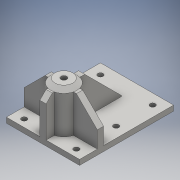
# Autodesk Inventor part: wing_sail_base_1
Saved by Autodesk Inventor 2016 (Build 200138000, 138)
## iProperties
Created: 2015-09-28
Part Number: wing_sail_base_1
Material: Generic
Document SubType Name: Modeling
Designer: Qiuyang
Density: 1 g/cm^3
Appearance: Default
Author: Qiuyang
Autodesk Inventor part; units mm, degrees
ref_plane "YZ Plane" through (0, 0, 0) normal (1, 0, 0) x (0, 1, 0)
ref_plane "XZ Plane" through (0, 0, 0) normal (0, 1, 0) x (-1, 0, 0)
ref_plane "XY Plane" through (0, 0, 0) normal (0, 0, 1) x (1, 0, 0)
sketch "Sketch1" plane through (0, 0, 0) normal (0, 0, 1) x (1, 0, 0)
  line L0 (0, 0) -> (70, 0)
  line L1 (70, 0) -> (70, 90)
  line L2 (70, 90) -> (0, 90)
  line L3 (0, 90) -> (0, 0)
  dimension "d0" = 70
  dimension "d1" = 90
  constraints: 8 end point, 2 parallel, 1 horizontal, 1 perpendicular
  measures "d0" distance of L2.end L1.end
  measures "d1" distance of L1.end L0.end
extrude "Extrusion1" add sketch "Sketch1" along normal blind 5
sketch "Sketch2" plane through (0, 0, 5) normal (0, 0, 1) x (1, 0, 0)
  circle A0 centre (35, 20) radius 12.5
  point P0 (0, 0)
  dimension "d4" = 25
  constraints: 1 centre point
  measures "d4" diameter of A0
extrude "Extrusion2" add sketch "Sketch2" along normal blind 40
sketch "Sketch3" plane through (35, 20, 45) normal (0, 0, 1) x (1, 0, 0)
  circle A0 centre (0, 0) radius 2.7
  point P0 (-35, -20)
  dimension "d7" = 5.4
  constraints: 1 centre point
  measures "d7" diameter of A0
extrude "Extrusion3" cut sketch "Sketch3" against normal blind 25
chamfer "Chamfer1" distance 4 angle 45 1 edges at (22.5, 20, 45) measured on face at (44.0861, 18.7875, 45)
sketch "Sketch4" plane through (0, 0, 5) normal (0, 0, 1) x (1, 0, 0)
  line L0 (0, 0) -> (70, 0) projected
  line L1 (32, 0) -> (38, 0)
  line L2 (38, 0) -> (38, 14)
  line L3 (38, 14) -> (32, 14)
  line L4 (32, 14) -> (32, 0)
  dimension "d13" = 6
  dimension "d14" = 14
  constraints: 8 end point, 2 parallel, 1 horizontal, 1 perpendicular, 1 point on line
  measures "d13" distance of L3.end L2.end
  measures "d14" distance of L2.end L1.end
extrude "Extrusion4" add sketch "Sketch4" along normal blind 36
chamfer "Chamfer2" distance 6 angle 45 1 edges at (35, 0, 41) measured on face at (35.3363, 2.5136, 41)
sketch "Sketch5" plane through (0, 0, 5) normal (0, 0, 1) x (1, 0, 0)
  line L0 (32, 72) -> (38, 72)
  line L1 (38, 72) -> (38, 27)
  line L2 (38, 27) -> (32, 27)
  line L3 (32, 27) -> (32, 72)
  line L4 (70, 0) -> (70, 90) projected
  line L5 (70, 23) -> (42, 23)
  line L6 (42, 23) -> (42, 17)
  line L7 (42, 17) -> (70, 17)
  line L8 (70, 17) -> (70, 23)
  line L9 (0, 90) -> (0, 0) projected
  line L10 (0, 23) -> (25.872, 23)
  line L11 (25.872, 23) -> (25.872, 17)
  line L12 (25.872, 17) -> (0, 17)
  line L13 (0, 17) -> (0, 23)
  dimension "d20" = 6
  dimension "d21" = 45
  dimension "d22" = 28
  dimension "d23" = 6
  constraints: 24 end point, 6 parallel, 4 point on line, 3 horizontal, 3 perpendicular
  measures "d20" distance of L1.end L2.end
  measures "d21" distance of L0.end L1.end
  measures "d22" distance of L7.end L6.end
  measures "d23" distance of L6.end L5.end
extrude "Extrusion5" add sketch "Sketch5" along normal blind 36
chamfer "Chamfer3" distance 20 angle 45 1 edges at (70, 20, 41) measured on face at (62.5, 20, 41)
chamfer "Chamfer4" distance 20 angle 45 1 edges at (0, 20, 41) measured on face at (7.5136, 20.3363, 41)
chamfer "Chamfer5" distance 35 angle 45 1 edges at (35, 72, 41) measured on face at (34, 72, 17)
sketch "Sketch6" plane through (0, 0, 5) normal (0, 0, 1) x (1, 0, 0)
  circle A0 centre (10, 7) radius 2.5
  circle A1 centre (60, 7) radius 2.5
  circle A2 centre (10, 80) radius 2.5
  circle A3 centre (60, 80) radius 2.5
  circle A4 centre (10, 45) radius 2.5
  circle A5 centre (60, 45) radius 2.5
  point P0 (0, 0)
  dimension "d35" = 5
  dimension "d36" = 5
  dimension "d37" = 5
  dimension "d38" = 5
  dimension "d39" = 5
  dimension "d40" = 5
  constraints: 6 centre point
  measures "d35" diameter of A0
  measures "d36" diameter of A1
  measures "d37" diameter of A2
  measures "d38" diameter of A3
  measures "d39" diameter of A4
  measures "d40" diameter of A5
extrude "Extrusion6" cut sketch "Sketch6" against normal blind 16
body "Solid1"
